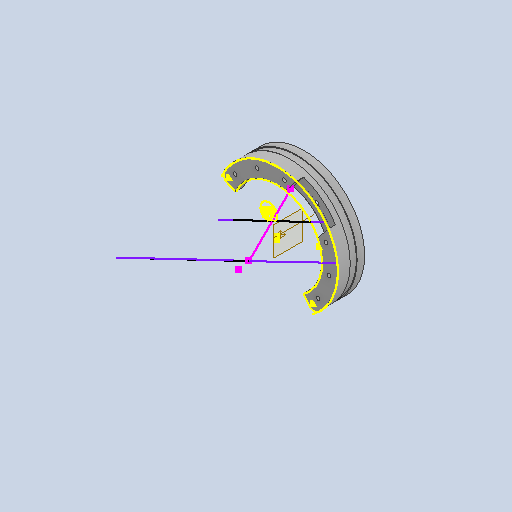
# Autodesk Inventor part: Anglerfish_Lightplate_Tosslink_base_flipped
Saved by Autodesk Inventor 2022 (Build 260153000, 153)
## iProperties
Created: 2022-07-21
Part Number: Anglerfish_Lightplate_Tosslink_base_flipped
Material: Generisch
Document SubType Name: Modeling
Designer: Muriel
Density: 1 g/cm^3
Appearance: Hellgrau
Author: Muriel
Autodesk Inventor part; units mm, degrees
ref_plane "XZ Plane" through (0, 0, 0) normal (0, 1, 0) x (-1, 0, 0)
ref_plane "XY Plane" through (0, 0, 0) normal (0, 0, 1) x (1, 0, 0)
ref_plane "Arbeitsebene4" through (0, 2.351, 3.7558) normal (1, 0, 0) x (0, 1, 0)
sketch "Skizze10" plane through (0, 2.351, 3.7558) normal (1, 0, 0) x (0, 1, 0)
  line L0 (-43.501, -12) -> (43.501, -12) projected
  line L1 (-43.501, -5.4848) -> (-43.501, -12)
  line L2 (-41.301, -11.7) -> (-41.301, -15.7)
  line L3 (-41.301, -15.7) -> (-46.301, -15.7)
  line L4 (-46.301, -15.7) -> (-46.301, 5)
  line L5 (-46.301, 5) -> (-34.301, 5)
  line L6 (-39.25, -1) -> (39.25, -1) projected
  line L7 (-34.301, 5) -> (-34.301, -1)
  line L8 (-34.301, -1) -> (-40.3733, -1)
  line L9 (-40.3733, -1) -> (-43.801, -4.4277)
  line L10 (-43.801, -4.4277) -> (-43.801, -12.3)
  line L11 (-43.801, -12.3) -> (-41.301, -11.7)
  line L12 (0, 9.14) -> (0, -19.84) projected
  line L13 (-46.301, -4.7072) -> (-45.7242, -4.7072)
  line L14 (-45.7242, -4.7072) -> (-45.7242, -9.988)
  line L15 (-45.7242, -9.988) -> (-46.301, -9.988)
  line L16 (-46.301, -9.988) -> (-46.301, -4.7072)
  point P0 (-2.351, -3.7558)
  point P1 (-41.301, -12)
  point P2 (-43.501, -11.793)
  point P3 (-42.551, -12)
  dimension "d36" = 4
  dimension "d37" = 5
  dimension "d38" = 135
  dimension "d39" = 0.3
  dimension "d40" = 2.5
  dimension "d41" = 6
  dimension "d42" = 12
  dimension "d43" = 0.6
  dimension "d56" = 0.3
  constraints: 28 end point, 5 perpendicular, 3 vertical, 2 horizontal, 2 parallel, 2 point on line, 1 other
  measures "d36" distance of L2.start L2.end
  measures "d37" distance of L2.end L3.end
  measures "d38" angle of L9 L8
  measures "d39" distance between parallel lines of L10 L1
  measures "d40" distance between parallel lines of L4 L10
  measures "d41" distance between parallel lines of L6 L5
  measures "d42" distance between parallel lines of L7 L4
  measures "d43" vertical distance of L10.end L2.start
  measures "d56" horizontal distance of L10.end L0.start
revolve "Umdrehung1" add sketch "Skizze10" angle 360 about axis through (0, 2.351, -8.2442) along (0, 0, -1) contours L0 L2 L3 L4 L15 L14 L13 L5 L7 L6 L8 L9 L10 L11
sketch "Skizze11" plane through (0, 2.351, 8.7558) normal (0, 0, 1) x (1, 0, 0)
  line L0 (-26.9619, -13.7457) -> (20.4346, 45.6645) projected
  line L1 (39.9774, 30.0736) -> (-7.4191, -29.3367) projected
  line L2 (-0.002, 0.0011) -> (27.4914, -37.256)
  circle A0 centre (0, 0) radius 46.301 projected
  line L3 (-0.002, 0.0011) -> (-42.4366, 18.5182)
  line L4 (0, 106.8921) -> (0, -174.7398) projected
  circle A1 centre (-0.002, 0.0011) radius 3.35 projected
  circle A2 centre (9.0619, 11.3655) radius 3 projected
  line L5 (9.0619, 11.3655) -> (-0.002, 0.0011)
  arc A3 (-12.3084, 5.3712) -> (7.9705, -10.8027) centre (-0.002, 0.0011) ccw
  circle A4 centre (6.6446, -5.3009) radius 1.9 projected
  point P0 (0, -2.351)
  dimension "d68" = 105
  dimension "d69" = 105
  constraints: 6 end point, 4 point on circle, 1 centre point, 1 coincident, 1 point on line
  measures "d68" angle of L2 L5
  measures "d69" angle of L5 L3
extrude "Extrusion9" cut sketch "Skizze11" against normal through all contours A3 L3 L0 | A3 L4 A0 L3 | L0 L3 A1 L4 A3 | A3 L1 L4 | L4 A1 L2 L1 A3 | L3 L4 A1 | L4 L2 A1 | L1 A3 L2 A0 L4 | L1 L2 A3 picked at (-0.274, -2.1983)
fillet "Rundung2" radius 5 2 edges at (-42.4366, 20.8692, -9.0882) (27.4914, -34.905, -9.0882)
sketch "Skizze13" plane through (0, 2.351, 8.7558) normal (0, 0, 1) x (0.6235512, 0.7817825, 0)
  arc A0 (7.4536, 6.6652) -> (0.6382, 9.9777) centre (6.3546, 13.0716) ccw projected
  arc A1 (7.4536, 6.6652) -> (0.6382, 9.9777) centre (0.0005, -0.002) ccw projected
  line L0 (10.2729, 12.2689) -> (9.4491, 10.3917) projected
  line L1 (9.4491, 10.3917) -> (9.2503, 10.479) projected
  arc A2 (9.2503, 10.479) -> (8.5915, 10.222) centre (9.0494, 10.0211) ccw projected
  line L2 (8.5915, 10.222) -> (7.9888, 8.8485) projected
  line L3 (7.9888, 8.8485) -> (2.1282, 11.4203) projected
  line L4 (2.1282, 11.4203) -> (2.7308, 12.7934) projected
  arc A3 (2.7308, 12.7934) -> (2.4729, 13.4531) centre (2.2732, 12.9948) ccw projected
  line L5 (2.4729, 13.4531) -> (2.3066, 13.5261) projected
  line L6 (2.3066, 13.5261) -> (3.1103, 15.3575) projected
  line L7 (3.1103, 15.3575) -> (3.2777, 15.2841) projected
  arc A4 (3.2777, 15.2841) -> (3.9366, 15.541) centre (3.4787, 15.7419) ccw projected
  line L8 (3.9366, 15.541) -> (4.2982, 16.3651) projected
  line L9 (4.2982, 16.3651) -> (5.6158, 16.879) projected
  line L10 (5.6158, 16.879) -> (9.6449, 15.1109) projected
  line L11 (9.6449, 15.1109) -> (10.2083, 13.7715) projected
  line L12 (10.2083, 13.7715) -> (9.8668, 12.9932) projected
  arc A5 (9.8668, 12.9932) -> (10.1237, 12.3344) centre (10.3246, 12.7923) ccw projected
  line L13 (10.1237, 12.3344) -> (10.2729, 12.2689) projected
  arc A6 (-8.8782, -33.1322) -> (-8.8782, 33.1322) centre (0, 0) ccw projected
  arc A7 (-6.4815, -45.8451) -> (-6.4817, 45.8451) centre (0, 0) ccw projected
  arc A8 (-6.4815, -45.8451) -> (-6.4817, 45.8451) centre (0, 0) ccw projected
  arc A9 (-8.8782, -33.1322) -> (-8.8782, 33.1322) centre (0, 0) ccw projected
  line L14 (34.8974, 14.5927) -> (15.9202, -24.4258) projected
  line L15 (-34.301, 0) -> (-134.7436, 48.8516)
  arc A10 (-8.8782, -33.1322) -> (-8.8782, 33.1322) centre (0, 0) ccw projected
  line L16 (33.7499, -6.1243) -> (-25.655, 22.768)
  line L17 (-134.7436, 48.8516) -> (-45.9256, 5.8844)
  arc A11 (-11.9838, -44.7233) -> (-11.9842, 44.7232) centre (0, 0) ccw projected
  arc A12 (-8.8782, -33.1322) -> (-8.8782, 33.1322) centre (0, 0) ccw projected
  line L18 (-25.655, 22.768) -> (-36.7661, 28.1432)
  line L19 (33.7499, -6.1243) -> (44.8864, -11.3575)
  arc A13 (-8.8782, -33.1322) -> (-8.8782, 33.1322) centre (0, 0) ccw projected
  line L20 (-34.301, 0) -> (33.12, -32.3551)
  line L21 (-8.8782, -33.1322) -> (-10.6112, -39.6004) projected
  line L22 (-10.6114, 39.6002) -> (-8.8782, 33.1322) projected
  line L23 (-8.8782, -33.1322) -> (-10.6112, -39.6004) projected
  line L24 (-10.6114, 39.6002) -> (-8.8782, 33.1322) projected
  arc A14 (-10.6112, -39.6004) -> (-6.4815, -45.8451) centre (-5.7815, -40.8944) ccw projected
  arc A15 (-6.4817, 45.8451) -> (-10.6114, 39.6002) centre (-5.7818, 40.8943) ccw projected
  arc A16 (-10.6112, -39.6004) -> (-6.4815, -45.8451) centre (-5.7815, -40.8944) ccw projected
  arc A17 (-6.4817, 45.8451) -> (-10.6114, 39.6002) centre (-5.7818, 40.8943) ccw projected
  point P0 (-1.838, -1.466)
  point P1 (28.2347, -19.4772)
  point P2 (-46.301, 0)
  point P3 (-46.301, 0)
  point P4 (9.2503, 10.479)
  point P5 (3.9366, 15.541)
  point P6 (9.8668, 12.9932)
  point P7 (10.1237, 12.3344)
  point P8 (33.7499, -6.1243)
  point P9 (-45.9256, 5.8844)
  point P10 (33.7499, -6.1243)
  point P11 (-25.655, 22.768)
  point P12 (21.4594, -26.7592)
  point P13 (-45.9529, 5.667)
  constraints: 12 end point, 6 point on circle, 3 point on line, 2 parallel, 1 perpendicular
ref_plane "Arbeitsebene6" through (-40.7561, -38.405, 2.7558) normal (0, 0, 1) x (0.9992339, 0.0391365, 0)
sketch "Skizze16" plane through (0, 2.351, 8.7558) normal (0, 0, 1) x (0.7817825, -0.6235512, 0)
  arc A0 (44.8655, -8.8196) -> (-44.8655, -8.8199) centre (0, 0) ccw projected
  circle A1 centre (0, 0) radius 40.3733
  arc A2 (38.9975, -10.4497) -> (-38.9975, -10.4499) centre (0, 0) ccw projected
  circle A3 centre (40.3733, 0) radius 1.4
  point P0 (1.466, -1.838)
  dimension "d70" = 2.8
  constraints: 2 centre point, 1 coincident, 1 point on circle
  measures "d70" diameter of A3
hole "Bohrung1" at (31.5631, -22.8238, 8.7558) direction (0, 0, -1) diameter 2.8 end through all
pattern_circular "Runde Anordnung1" count 12 over 360 about axis through (0, 2.351, 5.7558) along (0, 0, 1) of "Bohrung1"
sketch "Skizze17" plane through (0, 2.351, 8.7558) normal (0, 0, 1) x (0.7817825, -0.6235512, 0)
  line L0 (-12.5072, -27.5583) -> (-12.4988, 48.4417) projected
  line L1 (12.4928, -27.5611) -> (-12.5072, -27.5583) projected
  line L2 (12.5012, 48.4389) -> (12.4928, -27.5611) projected
  line L3 (-12.4988, 48.4417) -> (12.5012, 48.4389) projected
  line L4 (15.4925, -30.5614) -> (-15.5075, -30.558)
  line L5 (-15.5075, -30.558) -> (-15.4984, 51.442)
  line L6 (-15.4984, 51.442) -> (15.5016, 51.4386)
  line L7 (15.5016, 51.4386) -> (15.4925, -30.5614)
  point P0 (1.466, -1.838)
  dimension "d81" = 3
  constraints: 8 end point, 3 other
  measures "d81" distance between parallel lines of L2 L7
extrude "Extrusion14" cut sketch "Skizze17" against normal up to surface (5.5 mm away) contours L0 L3 L2 L1 | L4 L5 L6 L7
ref_plane "Arbeitsebene3" through (7.1263, -5.2789, 3.7558) normal (0, 0, 1) x (-0.6828675, 0.7305423, 0)
